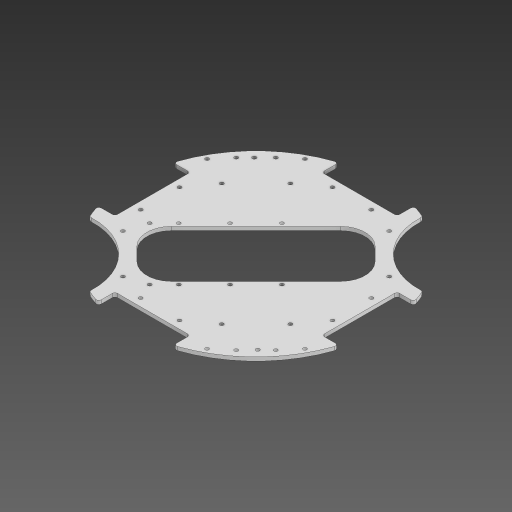
# Autodesk Inventor part: top
Saved by Autodesk Inventor 2023 (Build 270158000, 158)
## iProperties
Created: 2025-06-24
Part Number: top
Material: Типовые
Document SubType Name: Modeling
Designer: daa
Density: 1 g/cm^3
Appearance: По умолчанию
Author: daa
Autodesk Inventor part; units mm, degrees
ref_plane "YZ Plane" through (0, 0, 0) normal (1, 0, 0) x (0, 1, 0)
ref_plane "XZ Plane" through (0, 0, 0) normal (0, 1, 0) x (-1, 0, 0)
ref_plane "XY Plane" through (0, 0, 0) normal (0, 0, 1) x (1, 0, 0)
sketch "Эскиз1" plane through (0, 0, 0) normal (0, 1, 0) x (-1, 0, 0)
  line L0 (-79, -47.2724) -> (-79, 14.7276)
  line L1 (91.5447, -47.2724) -> (91.5447, 14.7276)
  line L2 (-79, -47.2724) -> (-93, -47.2724)
  line L3 (-79, 14.7276) -> (-93, 14.7276)
  line L4 (91.5447, -47.2724) -> (105.5447, -47.2724)
  line L5 (91.5447, 14.7276) -> (105.5447, 14.7276)
  line L6 (-24.7276, -101.5447) -> (37.2724, -101.5447)
  line L7 (-24.7276, 69) -> (37.2724, 69)
  line L8 (-24.7276, 69) -> (-24.7276, 83)
  line L9 (37.2724, 69) -> (37.2724, 83)
  line L10 (37.2724, -101.5447) -> (37.2724, -115.5447)
  line L11 (-24.7276, -101.5447) -> (-24.7276, -115.5447)
  arc A0 (-93, -47.2724) -> (-24.7276, -115.5447) centre (6.2724, -16.2724) ccw
  arc A1 (105.5447, 14.7276) -> (37.2724, 83) centre (6.2724, -16.2724) ccw
  arc A2 (-24.7276, 83) -> (-93, 14.7276) centre (6.2724, -16.2724) ccw
  arc A3 (37.2724, -115.5447) -> (105.5447, -47.2724) centre (6.2724, -16.2724) ccw
  dimension "d29" = 62
  dimension "d31" = 62
  dimension "d33" = 14
  dimension "d34" = 14
  dimension "d35" = 62
  dimension "d36" = 62
  dimension "d39" = 14
  dimension "d40" = 14
  constraints: 24 end point, 8 point on circle, 4 centre point, 4 horizontal, 3 parallel, 3 vertical, 2 point on line, 1 concentric
  measures "d29" distance of L0.start L0.end
  measures "d31" distance of L1.start L1.end
  measures "d33" distance of L0.end L3.end
  measures "d34" distance of L1.end L5.end
  measures "d35" distance of L6.start L6.end
  measures "d36" distance of L7.start L7.end
  measures "d39" distance of L7.start L8.end
  measures "d40" distance of L6.start L11.end
extrude "motor" add sketch "Эскиз1" along normal blind 3
sketch "Эскиз2" plane through (0, 3, 0) normal (0, 1, 0) x (1, 0, 0)
  arc A0 (24.7276, -83) -> (93, -14.7276) centre (-6.2724, 16.2724) ccw projected
  arc A1 (-37.2724, 115.5447) -> (-105.5447, 47.2724) centre (-6.2724, 16.2724) ccw projected
  circle A2 centre (-6.2724, 16.2724) radius 104
  line L0 (-6.2724, 16.2724) -> (-6.2724, -50.7276)
  arc A3 (-37.2724, 115.5447) -> (-105.5447, 47.2724) centre (-6.2724, 16.2724) ccw projected
  line L1 (-88.7917, -14.3063) -> (-40.8426, -62.2554)
  line L2 (-101.3809, -25.8032) -> (-48.3479, -78.8362)
  arc A4 (-105.5447, -14.7276) -> (-37.2724, -83) centre (-6.2724, 16.2724) ccw projected
  arc A5 (-48.3479, -78.8362) -> (-101.3809, -25.8032) centre (-98.035, -75.4903) ccw
  arc A6 (24.7276, -83) -> (93, -14.7276) centre (-6.2724, 16.2724) ccw projected
  line L3 (-79.8115, 89.8115) -> (67.2668, -57.2668)
  line L4 (24.3063, 98.7917) -> (72.2554, 50.8426)
  line L5 (35.8032, 111.3809) -> (88.8362, 58.3479)
  arc A7 (93, 47.2724) -> (24.7276, 115.5447) centre (-6.2724, 16.2724) ccw
  arc A8 (35.8032, 111.3809) -> (88.8362, 58.3479) centre (85.4903, 108.035) ccw
  line L6 (-91.5447, -14.7276) -> (-105.5447, -14.7276) projected
  arc A9 (-105.5447, -14.7276) -> (-101.3809, -25.8032) centre (-6.2724, 16.2724) ccw
  line L7 (-105.5447, -14.7276) -> (-80, -14.7276)
  point P0 (0, 0)
  point P1 (-6.2724, -50.7276)
  dimension "d181" = 208
  dimension "d190" = 67
  dimension "d205" = 75
  dimension "d207" = 17.0315
  dimension "d208" = 11.0756
  dimension "d209" = 104
  constraints: 14 end point, 10 point on circle, 7 symmetric about line, 5 centre point, 2 tangent, 1 point on line, 1 vertical, 2 other
  measures "d181" diameter of A2
  measures "d190" distance of L0.end L0.start
  measures "d205" distance of L2.start L2.end
  measures "d207" distance between parallel lines of L1 L2
  measures "d208" horizontal distance of A2.end L2.end
  measures "d209" radius of A9
extrude "ball" cut sketch "Эскиз2" against normal blind 3 contours A2 L2 | L2 A5 | L5 A2 | A8 L5
sketch "Эскиз3" plane through (0, 3, 0) normal (0, 1, 0) x (1, 0, 0)
  arc A0 (93, 47.2724) -> (24.7276, 115.5447) centre (-6.2724, 16.2724) ccw projected
  line L0 (-6.2724, 16.2724) -> (97.7276, 16.2724) construction
  line L1 (67.2668, 89.8115) -> (-62.5447, -40)
  circle A1 centre (70.5306, -44.2673) radius 1.5
  circle A2 centre (54.2672, -60.5308) radius 1.5
  circle A3 centre (41.3053, -71.6104) radius 1.5
  circle A4 centre (81.6104, -31.3053) radius 1.5
  arc A5 (24.7276, -83) -> (93, -14.7276) centre (-6.2724, 16.2724) ccw projected
  line L2 (-6.2724, 16.2724) -> (97.7276, 16.2724) construction
  line L3 (-79.8115, 89.8115) -> (67.2668, -57.2668)
  line L4 (-91.5447, 47.2724) -> (-91.5447, -14.7276) projected
  line L5 (-91.5447, 16.2724) -> (79, 16.2724)
  line L6 (24.7276, 101.5447) -> (-37.2724, 101.5447) projected
  line L7 (-6.2724, 101.5447) -> (-6.2724, -69)
  line L8 (-6.2724, 101.5447) -> (-6.2724, -69)
  line L9 (-91.5447, 47.2724) -> (-91.5447, -14.7276) projected
  arc A6 (24.7276, -83) -> (93, -14.7276) centre (-6.2724, 16.2724) ccw projected
  circle A7 centre (-66.812, 93.0753) radius 1.5
  circle A8 centre (-83.0755, 76.8119) radius 1.5
  circle A9 centre (-94.1551, 63.85) radius 1.5
  circle A10 centre (-53.85, 104.1551) radius 1.5
  point P0 (0, 0)
  point P1 (67.2668, -57.2668)
  point P2 (67.2668, -57.2668)
  point P3 (-105.5447, 47.2724)
  point P4 (-79.8115, 89.8115)
  point P5 (-79.8115, 89.8115)
  point P6 (-79.8115, 89.8115)
  dimension "d65" = 3
  dimension "d66" = 3
  dimension "d67" = 3
  dimension "d68" = 3
  dimension "d69" = 23
  dimension "d71" = 57
  dimension "d74" = -12.962
  dimension "d78" = 25.9614
  constraints: 14 end point, 8 centre point, 8 symmetric about line, 4 point on circle, 3 midpoint, 2 horizontal, 2 vertical, 1 point on line, 4 other
  measures "d65" diameter of A1
  measures "d66" diameter of A2
  measures "d67" diameter of A3
  measures "d68" diameter of A4
  measures "d69" distance of A2.centre A1.centre
  measures "d71" distance of A3.centre A4.centre
  measures "d74" vertical distance of A1.centre A4.centre
  measures "d78" vertical distance of A4.centre point (67.267, -57.267)
extrude "hand_mount" cut sketch "Эскиз3" against normal blind 10
sketch "Эскиз5" plane through (0, 3, 0) normal (0, 1, 0) x (1, 0, 0)
  circle A0 centre (29.7645, -47.992) radius 1.5
  circle A1 centre (58.0485, -19.7074) radius 1.5
  circle A2 centre (-6.2982, 16.355) radius 104
  arc A3 (-105.5447, -14.7276) -> (-99.04, -30.7083) centre (-6.2982, 16.355) ccw projected
  line L0 (-6.2982, 16.355) -> (97.7018, 16.355) construction
  line L1 (67.2409, 89.8941) -> (-79.8373, -57.1841)
  circle A4 centre (-70.6452, 52.4178) radius 1.5
  circle A5 centre (-42.3607, 80.7017) radius 1.5
  circle A6 centre (-44.9008, -54.7745) radius 1.5
  line L2 (-46.7704, -39.7817) -> (-62, -24)
  arc A7 (-53.253, -76.4953) -> (-99.04, -30.7083) centre (-88.8109, -66.2662) ccw projected
  line L3 (-62.7022, -40.049) -> (-61.1643, -38.511)
  line L4 (-61.1643, -38.511) -> (-44.8852, -38.511) construction
  line L5 (-61.1643, -38.511) -> (-44.9008, -54.7745)
  circle A8 centre (-77.4277, -22.2476) radius 1.5
  arc A9 (24.7276, -83) -> (93, -14.7276) centre (-6.2724, 16.2724) ccw projected
  line L6 (-6.2982, 16.355) -> (97.7785, 16.355) construction
  line L7 (67.2952, -57.2383) -> (-79.783, 89.8399)
  arc A10 (-37.2724, 115.5447) -> (-105.5447, 47.2724) centre (-6.2724, 16.2724) ccw projected
  circle A11 centre (64.8313, 54.9576) radius 1.5
  circle A12 centre (32.3044, 87.4845) radius 1.5
  point P0 (0, 0)
  dimension "d119" = 208
  dimension "d116" = 3
  dimension "d117" = 3
  dimension "d118" = 40
  dimension "d121" = 64.347
  dimension "d126" = 3
  dimension "d130" = 2.175
  dimension "d133" = 23
  constraints: 16 end point, 8 centre point, 5 symmetric about line, 4 point on circle, 3 horizontal, 2 point on line, 1 coincident, 9 other
  measures "d116" diameter of A0
  measures "d117" diameter of A1
  measures "d118" distance of A1.centre A0.centre
  measures "d121" vertical distance of L0.start A0.centre
  measures "d126" diameter of A6
  measures "d130" distance of L3.start L3.end
  measures "d133" distance of L3.end L5.end
extrude "Выдавливание5" cut sketch "Эскиз5" against normal blind 10 contours A0 | A1 | A4 | A5 | A6 | A8 | A11 | A12
sketch "Эскиз6" plane through (0, 3, 0) normal (0, 1, 0) x (1, 0, 0)
  circle A0 centre (-22.2724, 95.2947) radius 1.5
  circle A1 centre (9.7276, 95.2947) radius 1.5
  line L0 (24.7276, 115.5447) -> (24.7276, 101.5447) projected
  line L1 (24.7276, 101.5447) -> (-37.2724, 101.5447) projected
  circle A2 centre (-22.2724, -62.75) radius 1.5
  circle A3 centre (9.7276, -62.75) radius 1.5
  circle A4 centre (-85.2947, 32.2724) radius 1.5
  circle A5 centre (-85.2947, 0.2724) radius 1.5
  circle A6 centre (72.75, 32.2724) radius 1.5
  circle A7 centre (72.75, 0.2724) radius 1.5
  point P0 (0, 0)
  point P1 (24.7276, -69)
  point P2 (-37.2724, -69)
  point P3 (-91.5447, -14.7276)
  point P4 (-91.5447, 47.2724)
  point P5 (79, 47.2724)
  point P6 (79, -14.7276)
  dimension "d135" = 3
  dimension "d136" = 3
  dimension "d137" = 32
  dimension "d138" = 15
  dimension "d139" = 6.25
  dimension "d140" = 3
  dimension "d141" = 3
  dimension "d142" = 6.25
  dimension "d143" = 32
  dimension "d144" = 15
  dimension "d145" = 6.25
  dimension "d146" = 6.25
  dimension "d147" = 3
  dimension "d148" = 3
  dimension "d149" = 32
  dimension "d150" = 15
  dimension "d151" = 6.25
  dimension "d152" = 6.25
  dimension "d153" = 3
  dimension "d154" = 3
  dimension "d155" = 32
  dimension "d156" = 15
  dimension "d157" = 6.25
  dimension "d158" = 6.25
  constraints: 8 centre point
  measures "d135" diameter of A0
  measures "d136" diameter of A1
  measures "d137" distance of A1.centre A0.centre
  measures "d138" distance from line of L0 A1.centre
  measures "d139" distance from line of L1 A1.centre
  measures "d140" diameter of A2
  measures "d141" diameter of A3
  measures "d142" distance from line of L1 A0.centre
  measures "d143" distance of A2.centre A3.centre
  measures "d144" horizontal distance of point (24.728, -69) A3.centre
  measures "d145" vertical distance of point (24.728, -69) A3.centre
  measures "d146" vertical distance of point (-37.272, -69) A2.centre
  measures "d147" diameter of A4
  measures "d148" diameter of A5
  measures "d149" distance of A5.centre A4.centre
  measures "d150" vertical distance of A5.centre point (-91.545, -14.728)
  measures "d151" horizontal distance of A5.centre point (-91.545, -14.728)
  measures "d152" horizontal distance of A4.centre point (-91.545, 47.272)
  measures "d153" diameter of A6
  measures "d154" diameter of A7
  measures "d155" distance of A7.centre A6.centre
  measures "d156" vertical distance of point (79, 47.272) A6.centre
  measures "d157" horizontal distance of point (79, -14.728) A7.centre
  measures "d158" horizontal distance of point (79, 47.272) A6.centre
extrude "Выдавливание6" cut sketch "Эскиз6" against normal blind 10
fillet "Сопряжение1" radius 2 16 edges at (93, 1.5, -47.2724) (24.7276, 1.5, -115.5447) (24.7276, 1.5, -101.5447) (-37.2724, 1.5, -101.5447) (-37.2724, 1.5, -115.5447) (-105.5447, 1.5, -47.2724) (-91.5447, 1.5, -47.2724) (-91.5447, 1.5, 14.7276) (-105.5447, 1.5, 14.7276) (-37.2724, 1.5, 83) (-37.2724, 1.5, 69) (24.7276, 1.5, 69) (24.7276, 1.5, 83) (93, 1.5, 14.7276) (79, 1.5, 14.7276) (79, 1.5, -47.2724)
fillet "Сопряжение4" radius 2 4 edges at (-101.3809, 1.5, 25.8032) (-48.3479, 1.5, 78.8362) (35.8032, 1.5, -111.3809) (88.8362, 1.5, -58.3479)
sketch "Эскиз8" plane through (0, 3, 0) normal (0, 1, 0) x (1, 0, 0)
  circle A0 centre (-75.6509, 84.2365) radius 1.6
  circle A1 centre (62.8514, -51.4283) radius 1.6
  circle A2 centre (-83.0755, 76.8119) radius 1.5
  circle A3 centre (-83.0755, 76.8119) radius 1.5 projected
  line L0 (-83.0755, 76.8119) -> (-75.6509, 84.2365)
  line L1 (-83.0755, 76.8119) -> (-72.5755, 76.8119) construction
  circle A4 centre (54.2672, -60.5308) radius 1.5
  circle A5 centre (54.2672, -60.5308) radius 1.5 projected
  line L2 (54.2672, -60.5308) -> (67.7672, -60.5308) construction
  circle A6 centre (70.5306, -44.2673) radius 1.5
  circle A7 centre (70.5306, -44.2673) radius 1.5 projected
  line L3 (70.5306, -44.2673) -> (62.8514, -51.4283)
  line L4 (70.5306, -44.2673) -> (81.0306, -44.2673) construction
  point P0 (0, 0)
  dimension "d211" = 3.2
  dimension "d212" = 3.2
  dimension "d213" = 3
  dimension "d214" = 10.5
  dimension "d215" = 45
  dimension "d216" = 3
  dimension "d221" = 3
  dimension "d222" = 10.5
  dimension "d223" = 137
  constraints: 10 end point, 5 centre point, 3 concentric, 3 horizontal, 2 coincident, 2 equal length
  measures "d211" diameter of A0
  measures "d212" diameter of A1
  measures "d213" diameter of A2
  measures "d214" distance of L0.start L0.end
  measures "d215" angle of L1 L0
  measures "d216" diameter of A4
  measures "d221" diameter of A6
  measures "d222" distance of L3.start L3.end
  measures "d223" angle of L3 L4
extrude "Выдавливание7" cut sketch "Эскиз8" against normal blind 10 contours A0 | A1
sketch "Эскиз9" plane through (0, 3, 0) normal (0, 1, 0) x (1, 0, 0)
  line L0 (-38.87, 27.5154) -> (-17.5154, 48.87)
  line L1 (-17.5154, 48.87) -> (26.3253, 5.0294)
  line L2 (26.3253, 5.0294) -> (4.9706, -16.3253)
  line L3 (4.9706, -16.3253) -> (-38.87, 27.5154)
  circle A0 centre (-6.2724, 16.2724) radius 104
  arc A1 (-39.9194, 114.679) -> (-104.679, 49.9194) centre (-6.2724, 16.2724) ccw projected
  circle A2 centre (-17.5154, 48.87) radius 1.5
  circle A3 centre (-38.87, 27.5154) radius 1.5
  circle A4 centre (4.9706, -16.3253) radius 1.5
  circle A5 centre (26.3253, 5.0294) radius 1.5
  point P0 (0, 0)
  dimension "d224" = 30.2
  dimension "d225" = 62
  dimension "d226" = 208
  dimension "d227" = 15.1
  dimension "d229" = 31
  dimension "d230" = 3
  dimension "d231" = 3
  dimension "d232" = 3
  dimension "d233" = 3
  constraints: 8 end point, 5 centre point, 4 coincident, 2 parallel, 1 concentric, 1 perpendicular
  measures "d224" distance of L1.end L2.end
  measures "d225" distance of L0.end L1.end
  measures "d226" diameter of A0
  measures "d227" distance from line of L1 A0.centre
  measures "d229" distance from line of L2 A0.centre
  measures "d230" diameter of A2
  measures "d231" diameter of A3
  measures "d232" diameter of A4
  measures "d233" diameter of A5
extrude "Выдавливание8" cut sketch "Эскиз9" against normal blind 10 contours L3 A3 L0 | L0 A3 L3 | A2 L1 L0 | L0 L1 A2 | A4 L2 L3 | L3 L2 A4 | A5 L2 L1 | L1 L2 A5
sketch "Эскиз10" plane through (0, 3, 0) normal (0, 1, 0) x (1, 0, 0)
  circle A0 centre (-6.2724, 16.2719) radius 104.0005
  arc A1 (-39.9194, 114.679) -> (-104.679, 49.9194) centre (-6.2724, 16.2724) ccw projected
  line L0 (-60.0125, 6.3729) -> (-72.0333, -5.648)
  line L1 (-72.0333, -5.648) -> (-28.1927, -49.4886)
  line L2 (-28.1927, -49.4886) -> (-16.1718, -37.4678)
  line L3 (-16.1718, -37.4678) -> (-60.0125, 6.3729)
  circle A2 centre (-60.0125, 6.3729) radius 1.5
  circle A3 centre (-72.0333, -5.648) radius 1.5
  circle A4 centre (-16.1718, -37.4678) radius 1.5
  circle A5 centre (-28.1927, -49.4886) radius 1.5
  point P0 (0, 0)
  dimension "d248" = 17
  dimension "d249" = 62
  dimension "d250" = 9.899
  dimension "d251" = 45
  dimension "d252" = 3
  dimension "d253" = 3
  dimension "d254" = 3
  dimension "d255" = 3
  constraints: 8 end point, 5 centre point, 4 coincident, 2 parallel, 1 perpendicular, 1 tangent
  measures "d248" distance of L2.end L1.end
  measures "d249" distance of L1.end L0.end
  measures "d250" vertical distance of L0.start A0.centre
  measures "d251" distance from line of L3 A1.centre
  measures "d252" diameter of A2
  measures "d253" diameter of A3
  measures "d254" diameter of A4
  measures "d255" diameter of A5
extrude "Выдавливание9" cut sketch "Эскиз10" against normal blind 10 contours L3 A2 L0 | L0 A2 L3 | A3 L1 L0 | L0 L1 A3 | A4 L2 L3 | L3 L2 A4 | A5 L2 L1 | L1 L2 A5
sketch "Эскиз12" plane through (0, 3, 0) normal (0, 1, 0) x (1, 0, 0)
  line L0 (-49.8565, -38.2721) -> (-60.8166, -27.3119)
  line L1 (-60.8166, 0.9723) -> (9.0278, 70.8168)
  line L2 (37.3121, 70.8168) -> (48.2723, 59.8566)
  line L3 (48.2723, 31.5724) -> (-21.5722, -38.2721)
  circle A0 centre (-6.2724, 16.2724) radius 104
  arc A1 (27.3747, -82.1343) -> (92.1343, -17.3747) centre (-6.2724, 16.2724) ccw projected
  arc A2 (48.2723, 31.5724) -> (48.2723, 59.8566) centre (34.1301, 45.7145) ccw
  arc A3 (37.3121, 70.8168) -> (9.0278, 70.8168) centre (23.17, 56.6747) ccw
  arc A4 (-60.8166, 0.9723) -> (-60.8166, -27.3119) centre (-46.6745, -13.1698) ccw
  arc A5 (-49.8565, -38.2721) -> (-21.5722, -38.2721) centre (-35.7144, -24.13) ccw
  point P0 (0, 0)
  point P1 (-35.7144, -52.4142)
  point P2 (23.17, 84.9589)
  point P3 (-74.9588, -13.1698)
  point P4 (62.4144, 45.7145)
  dimension "d256" = 55.5
  dimension "d257" = 138.775
  dimension "d258" = 208
  dimension "d259" = 29.442
  dimension "d260" = -29.4422
  dimension "d261" = 20
  constraints: 9 tangent, 8 end point, 8 point on circle, 8 point on line, 5 centre point, 3 equal radius, 2 parallel, 1 perpendicular
  measures "d256" distance of point (23.17, 84.959) point (62.414, 45.715)
  measures "d257" distance of point (-74.959, -13.17) point (23.17, 84.959)
  measures "d258" diameter of A0
  measures "d259" horizontal distance of A1.centre point (-35.714, -52.414)
  measures "d260" vertical distance of point (-74.959, -13.17) A1.centre
  measures "d261" radius of A2
extrude "Выдавливание10" cut sketch "Эскиз12" against normal blind 10 contours L0 A4 L1 A3 L2 A2 L3 A5
